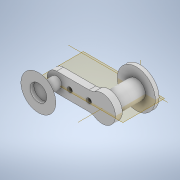
# Autodesk Inventor part: Herramientav2
Saved by Autodesk Inventor 2022 (Build 260153000, 153)
## iProperties
Created: 2022-11-16
Part Number: Herramientav2
Material: Genérico
Document SubType Name: Modeling
Designer: javie
Density: 1 g/cm^3
Appearance: Valor por defecto
Author: javie
Autodesk Inventor part; units mm, degrees
ref_plane "YZ Plane" through (0, 0, 0) normal (1, 0, 0) x (0, 1, 0)
ref_plane "XZ Plane" through (0, 0, 0) normal (0, 1, 0) x (-1, 0, 0)
ref_plane "XY Plane" through (0, 0, 0) normal (0, 0, 1) x (1, 0, 0)
sketch "Boceto2" plane through (0, 0, 0) normal (0, 0, 1) x (1, 0, 0)
  circle A0 centre (0, 0) radius 25
  dimension "d0" = 50
  constraints: 1 centre point, 1 coincident
  measures "d0" diameter of A0
extrude "Extrusión1" add sketch "Boceto2" along normal blind 5
sketch "Boceto3" plane through (0, 0, 5) normal (0, 0, 1) x (1, 0, 0)
  circle A0 centre (0, 0) radius 12
  dimension "d3" = 24
  constraints: 1 centre point, 1 coincident
  measures "d3" diameter of A0
extrude "Extrusión2" add sketch "Boceto3" along normal blind 36
sketch "Boceto4" plane through (0, 0, 41) normal (0, 0, 1) x (1, 0, 0)
  line L0 (-17.3205, 12.5) -> (-60, 12.5)
  line L1 (-60, -12.5) -> (-17.3205, -12.5)
  arc A0 (-60, 12.5) -> (-60, -12.5) centre (-60, 0) ccw
  arc A1 (-9.3264, -14.8077) -> (-9.3264, 14.8077) centre (0, 0) ccw
  arc A2 (-17.3205, 12.5) -> (-9.3264, 14.8077) centre (-17.3205, 27.5) ccw
  arc A3 (-9.3264, -14.8077) -> (-17.3205, -12.5) centre (-17.3205, -27.5) ccw
  circle A4 centre (0, 0) radius 8.1
  circle A5 centre (-42.5, 0) radius 3.25
  circle A6 centre (-17.3205, 0) radius 3.25
  circle A7 centre (-60, 0) radius 7
  point P0 (0, 0)
  point P1 (-12.2474, 12.5)
  point P2 (-12.2474, -12.5)
  point P3 (-17.175, 19.5112)
  constraints: 10 point on circle, 8 centre point, 4 end point, 4 tangent, 2 coincident, 2 point on line, 1 equal radius, 1 horizontal, 1 parallel
extrude "Extrusión3" add sketch "Boceto4" along normal blind 9 contours A2 A1 A3 L1 A0 L0 | A4
ref_plane "Plano de trabajo1" through (-60, 0, 41) normal (0, 1, 0) x (1, 0, 0)
sketch "Boceto6" plane through (-60, 0, 41) normal (0, 1, 0) x (1, 0, 0)
  line L0 (7, -9) -> (7, 0)
  line L1 (7, 0) -> (-7, 0)
  line L2 (-7, 0) -> (-7, -9)
  line L3 (-7, -9) -> (-7, -22)
  line L4 (7, -9) -> (7, -22)
  line L5 (-23, -33) -> (23, -33)
  line L6 (-7, -22) -> (-23, -33)
  line L7 (7, -22) -> (23, -33)
  line L8 (0, 5.1032) -> (0, -35.579)
  point P0 (60, 41)
  point P1 (0, 0)
  point P2 (0, -33)
  dimension "d8" = 14
  dimension "d9" = 9
  dimension "d10" = 13
  dimension "d11" = 13
  dimension "d12" = 46
  dimension "d13" = 11
  constraints: 18 end point, 2 vertical, 1 horizontal, 1 parallel
  measures "d8" distance of L1.end L0.end
  measures "d9" distance of L1.end L2.end
  measures "d10" distance of L2.end L3.end
  measures "d11" distance of L0.start L4.end
  measures "d12" distance of L5.start L5.end
  measures "d13" distance from line of L5 L4.end
revolve "Revolución1" add sketch "Boceto6" angle 360 about axis through (-60, 0, 35.8968) along (0, 0, 1) contours L4 L7 L5 L8 L1 L0
sketch "Boceto7" plane through (-60, 0, 74) normal (0, 0, 1) x (1, 0, 0)
  circle A0 centre (0, 0) radius 23 projected
  circle A1 centre (0, 0) radius 11
  point P0 (60, 0)
  dimension "d15" = 22
  constraints: 1 centre point, 1 coincident
  measures "d15" diameter of A1
extrude "Extrusión4" cut sketch "Boceto7" against normal blind 5 contours A1
